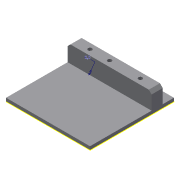
# Autodesk Inventor part: misc_hand_stand
Saved by Autodesk Inventor 2014 (Build 180170000, 170)
## iProperties
Created: 2015-08-17
Part Number: misc_hand_stand
Material: Generic
Document SubType Name: Modeling
Designer: Martin
Density: 1 g/cm^3
Appearance: Default
Author: Martin
Autodesk Inventor part; units mm, degrees
ref_plane "YZ Plane" through (0, 0, 0) normal (1, 0, 0) x (0, 1, 0)
ref_plane "XZ Plane" through (0, 0, 0) normal (0, 1, 0) x (-1, 0, 0)
ref_plane "XY Plane" through (0, 0, 0) normal (0, 0, 1) x (1, 0, 0)
sketch "Sketch1" plane through (0, 0, 0) normal (0, 0, 1) x (1, 0, 0)
  line L0 (-52.5, 0) -> (52.5, 0) projected
  line L1 (0, -52.5) -> (0, 52.5) projected
  line L2 (-37.5, -37.5) -> (37.5, -37.5)
  line L3 (37.5, -37.5) -> (37.5, 37.5)
  line L4 (37.5, 37.5) -> (-37.5, 37.5)
  line L5 (-37.5, 37.5) -> (-37.5, -37.5)
  line L6 (-37.5, -37.5) -> (37.5, 37.5) construction
  line L7 (37.5, -37.5) -> (-37.5, 37.5) construction
  point P0 (0, 0)
  dimension "d0" = 75
  dimension "d1" = 75
  constraints: 12 end point, 2 midpoint, 2 parallel, 1 horizontal, 1 perpendicular
  measures "d0" distance of L3.end L4.end
  measures "d1" distance of L2.end L3.end
extrude "Extrusion1" add sketch "Sketch1" along normal blind 3
sketch "Sketch2" plane through (0, 0, 3) normal (0, 0, 1) x (1, 0, 0)
  line L0 (37.5, -37.5) -> (37.5, 37.5) projected
  line L1 (37.5, 37.5) -> (-37.5, 37.5) projected
  line L2 (37.5, 17.5) -> (37.5, 27.5)
  line L3 (37.5, 27.5) -> (-37.5, 27.5)
  line L4 (-37.5, 27.5) -> (-37.5, 17.5)
  line L5 (-37.5, 17.5) -> (37.5, 17.5)
  point P0 (0, 0)
  dimension "d4" = 10
  dimension "d5" = 10
  constraints: 8 end point, 2 parallel, 2 point on line, 1 perpendicular
  measures "d4" distance between parallel lines of L1 L3
  measures "d5" distance between parallel lines of L5 L3
extrude "Extrusion2" add sketch "Sketch2" along normal blind 15
chamfer "Chamfer1" distance 2.5 angle 45 2 edges at (37.5, 22.5, 18) (-37.5, 22.5, 18)
sketch "Sketch3" plane through (0, 0, 18) normal (0, 0, 1) x (1, 0, 0)
  line L0 (-35, 17.5) -> (-35, 27.5) projected
  line L1 (35, 27.5) -> (35, 17.5) projected
  line L2 (-35, 22.5) -> (35, 22.5) construction
  circle A0 centre (-5, 22.5) radius 1.75
  circle A1 centre (-22.5, 22.5) radius 1.75
  line L3 (0, -52.5) -> (0, 52.5) projected
  circle A2 centre (22.5, 22.5) radius 1.75
  point P0 (0, 0)
  dimension "d11" = 45
  dimension "d12" = 17.5
  dimension "d13" = 5
  dimension "d14" = 3.5
  constraints: 3 centre point, 3 point on line, 2 end point, 2 equal radius, 2 midpoint
  measures "d11" distance of A2.centre A1.centre
  measures "d12" distance of A0.centre A1.centre
  measures "d13" distance from line of L3 A0.centre
  measures "d14" diameter of A2
extrude "Extrusion3" cut sketch "Sketch3" against normal through all
sketch "Sketch4" plane through (0, 0, 0) normal (0, 0, -1) x (-1, 0, 0)
  circle A0 centre (22.5, 22.5) radius 1.75 projected
  circle A1 centre (5, 22.5) radius 1.75 projected
  circle A2 centre (-22.5, 22.5) radius 1.75 projected
  line L0 (37.5, -37.5) -> (-37.5, -37.5) projected
  line L1 (37.5, 37.5) -> (37.5, -37.5) projected
  line L2 (-37.5, 37.5) -> (37.5, 37.5) projected
  line L3 (-37.5, -37.5) -> (-37.5, 37.5) projected
  circle A3 centre (-22.5, 22.5) radius 3.25
  circle A4 centre (5, 22.5) radius 3.25
  circle A5 centre (22.5, 22.5) radius 3.25
  point P0 (0, 0)
  dimension "d17" = 6.5
  constraints: 3 centre point, 3 coincident, 2 equal radius
  measures "d17" diameter of A5
body "Solid1"
